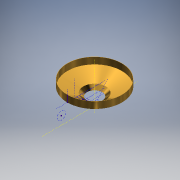
# Autodesk Inventor part: objective_shield_2
Saved by Autodesk Inventor 2018 (Build 220112000, 112)
## iProperties
Created: 2017-08-25
Part Number: objective_shield_2
Material: Brass, Soft Yellow
Document SubType Name: Sheet Metal
Designer: richp
Density: 8.47 g/cm^3
Appearance: Brass - Satin
Sheet Metal Rule: Default
Mass: 3.01003 g
Surface Area: 40.2715 cm^2
Volume: 0.355375 cm^3
cone1_major_rad: 0.819 in
cone1_minor_rad: 0.330 in
cone2_hieght: 0.080 in
cone2_minor_rad: 0.225 in
cone1_height: 0.170 in
ring_hieght: 0.200 in
Author: richp
Autodesk Inventor part; units mm, degrees
ref_plane "YZ Plane" through (0, 0, 0) normal (1, 0, 0) x (0, 1, 0)
ref_plane "XZ Plane" through (0, 0, 0) normal (0, 1, 0) x (-1, 0, 0)
ref_plane "XY Plane" through (0, 0, 0) normal (0, 0, 1) x (1, 0, 0)
sketch "Sketch1" plane through (0, 0, 0) normal (1, 0, 0) x (0, 1, 0)
  line L0 (-5.1799, 0) -> (31.0792, 0) construction
  line L1 (0, -33.1988) -> (0, 40.25) construction
  line L2 (0, 0) -> (13, 9.7962) construction
  line L3 (0, 0) -> (13, -9.7962) construction
  line L4 (3.35, 2.6) -> (0.75, 2.6) construction
  line L5 (0.75, 2.6) -> (0.75, -2.6) construction
  line L6 (0.75, -2.6) -> (3.35, -2.6) construction
  line L7 (3.35, -2.6) -> (3.35, 2.6) construction
  line L8 (4.874, 11.4005) -> (4.874, -12.8161) construction
  line L9 (7.922, 11.2583) -> (7.922, -12.1988) construction
  circle A0 centre (6.398, 25.4) radius 3.175 construction
  line L10 (12.748, 29.7573) -> (12.748, -6.0773) construction
  line L11 (13, -8.155) -> (13, 15.6322) construction
  line L12 (12.748, 20.81) -> (8.422, 8.3886)
  line L13 (13, 11.8384) -> (4.874, 5.715) construction
  line L14 (12.9363, 20.81) -> (12.8744, 20.6322) construction
  line L15 (12.748, 20.81) -> (21.6933, 20.81) construction
  line L16 (12.9363, 20.81) -> (12.748, 20.81)
  line L17 (8.6773, 8.581) -> (8.422, 8.3886)
  line L18 (0, 3.81) -> (0, -3.81) construction
  line L19 (0, 3.81) -> (13, 13.6062) construction
  line L20 (13, 15.6322) -> (25.8994, 15.6322) construction
  line L21 (17.828, 20.81) -> (17.828, 20.6322)
  line L22 (17.828, 20.6322) -> (12.8744, 20.6322)
  line L23 (17.828, 20.81) -> (12.9363, 20.81)
  line L24 (12.8744, 20.6322) -> (8.6773, 8.581)
  line L25 (4.874, 5.715) -> (7.922, 8.763) construction
  line L26 (5, -22.7061) -> (5, -16.8713)
  line L27 (8.422, 8.3886) -> (8.422, 7.251) construction
  line L28 (8.422, 7.251) -> (3.35, 3.429) construction
  line L29 (6.398, 5.7258) -> (12.748, 13.6802) construction
  dimension "d0" = 37
  dimension "d1" = 13
  dimension "d2" = 2.6
  dimension "d3" = 5.2
  dimension "d4" = 0.75
  dimension "d5" = 1.524
  dimension "d6" = 3.048
  dimension "d7" = 6.35
  dimension "d8" = 1.524
  dimension "d9" = 25.4
  dimension "d10" = 3.175
  dimension "cone1_major_rad" = 20.81
  dimension "d13" = 0.5
  dimension "d15" = 5.715
  dimension "d17" = 0.1778
  dimension "d19" = 7.62
  dimension "d21" = 5.1778
  dimension "d22" = 0.1778
  dimension "ring_hieght" = 5.08
  dimension "cone1_minor_rad" = 8.3886
  dimension "cone1_height" = 4.326
  dimension "d26" = 45
  dimension "d27" = 5
  dimension "d29" = 2.286
  dimension "d30" = 7.251
  dimension "d31" = 13.6802
  dimension "cone2_minor_rad" = 5.7258
  dimension "d33" = 6.35
  dimension "d34" = 8.581
  dimension "cone2_hieght" = 2.024
  constraints: 56 end point, 16 point on line, 7 parallel, 7 vertical, 3 horizontal, 3 perpendicular, 2 symmetric about line, 1 centre point, 1 collinear, 1 vertical alignment, 1 other
  measures "d0" angle of L0 L2
  measures "d1" distance from line of L1 L2.end
  measures "d2" distance between parallel lines of L5 L7
  measures "d3" distance between parallel lines of L4 L6
  measures "d4" distance between parallel lines of L1 L5
  measures "d5" distance between parallel lines of L7 L8
  measures "d6" distance between parallel lines of L8 L9
  measures "d7" diameter of A0
  measures "d8" distance from line of L8 A0.centre
  measures "d9" vertical distance of A0.centre L2.start
  measures "d10" distance edge to line of A0 L10
  measures "cone1_major_rad" distance from line of L0 L12.start
  measures "d13" distance from line of L9 L12.end
  measures "d15" distance from line of L0 L13.end
  measures "d17" distance between parallel lines of L12 L14
  measures "d19" distance of L18.start L18.end
  measures "d21" distance between parallel lines of L15 L20
  measures "d22" distance between parallel lines of L15 L22
  measures "ring_hieght" horizontal distance of L21.end L12.start
  measures "cone1_minor_rad" distance from line of L0 L12.end
  measures "cone1_height" distance from line of L12.end L10
  measures "d26" angle of L8 L25
  measures "d27" distance between parallel lines of L1 L26
  measures "d29" vertical distance of L28.end L13.end
  measures "d30" distance from line of L0 L27.end
  measures "d31" distance from line of L0 L29.end
  measures "cone2_minor_rad" distance from line of L0 L29.start
  measures "d33" distance from line of L10 L29.start
  measures "d34" distance from line of L0 L17.start
  measures "cone2_hieght" horizontal distance of L12.end L29.start
revolve "Revolution1" add sketch "Sketch1" angle 360 about axis through (0, -10, 0) along (0, 1, 0)
sketch "Sketch2" plane through (0, 0, 0) normal (1, 0, 0) x (0, 1, 0)
  line L0 (8.6773, 8.581) -> (8.422, 8.3886) projected
  line L1 (0, 0) -> (13, 9.7962) construction
  line L2 (8.422, 8.3886) -> (8.422, 6.3464)
  line L3 (8.6773, 8.581) -> (8.6773, 6.5388)
  line L4 (8.422, 6.3464) -> (8.6773, 6.5388)
  line L5 (-5.1799, 0) -> (31.0792, 0) construction
  constraints: 6 end point, 2 point on line, 1 parallel, 1 vertical
revolve "Revolution2" [suppressed]
sketch "Sketch4" plane through (0, 0, 0) normal (1, 0, 0) x (0, 1, 0)
  line L0 (6.398, 5.7258) -> (12.748, 13.6802) construction
  line L1 (8.6773, 8.581) -> (6.398, 5.7258)
  line L2 (8.5383, 8.6919) -> (6.259, 5.8368)
  line L3 (6.398, 5.7258) -> (6.259, 5.8368)
  line L4 (8.6773, 8.581) -> (8.5383, 8.6919)
  line L5 (-5.1799, 0) -> (31.0792, 0) construction
  point P0 (0, 0)
  dimension "d36" = 0.1778
  constraints: 8 end point, 2 perpendicular, 1 parallel
  measures "d36" distance between parallel lines of L0 L2
revolve "Revolution3" add sketch "Sketch4" angle 360 about axis through (0, -5.1799, 0) along (0, 1, 0)
equation "\"d8\" = 0.5 * d6"
equation "\"cone1_major_rad\" = 0.5 * main_aperture_diameter"
equation "\"d15\" = 0.5 * headplate_aperture_diameter"
equation "\"d19\" = fov_diameter"
equation "\"d21\" = 0.5 * EO_20x_diameter - 0.5 * E0_20x_front_aperture_diameter + d17"
equation "\"d22\" = d17"
equation "\"d36\" = d17"
equation "\"BendRadius\" = Thickness"
equation "\"BendReliefWidth\" = Thickness"
equation "\"BendReliefDepth\" = 0.5 * Thickness"
equation "\"CornerReliefSize\" = 4 * Thickness"
equation "\"MinimumRemnant\" = 2 * Thickness"
equation "\"TransitionRadius\" = BendRadius"
equation "\"JacobiRadiusSize\" = Thickness"
equation "\"GapSize\" = Thickness"
equation "\"main_aperture_diameter\" = 41.62"
equation "\"headplate_aperture_diameter\" = 11.43"
equation "\"fov_diameter\" = 7.62"
equation "\"EO_20x_diameter\" = 33.999932"
equation "\"E0_20x_front_aperture_diameter\" = 24.000003"
equation "\"Thickness\" = 3.048"
body "Solid1"
